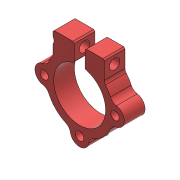
# Autodesk Inventor part: 16_022_TIBIA_PIPE_CLAMPER_R1
Saved by Autodesk Inventor 2021.2 (Build 252289000, 289)
## iProperties
Created: 2018-07-20
Part Number: 16_022_TIBIA_PIPE_CLAMPER_R1
Material: アルミニウム 6061
Document SubType Name: Modeling
Designer: student
Density: 2.7 g/cm^3
Appearance: 滑らか - 赤
Mass: 0.864961 g
Surface Area: 6.24289 cm^2
Volume: 0.320356 cm^3
Author: student
Autodesk Inventor part; units mm, degrees
ref_plane "YZ Plane" through (0, 0, 0) normal (1, 0, 0) x (0, 1, 0)
ref_plane "XZ Plane" through (0, 0, 0) normal (0, 1, 0) x (-1, 0, 0)
ref_plane "XY Plane" through (0, 0, 0) normal (0, 0, 1) x (1, 0, 0)
sketch "スケッチ1" plane through (0, 0, 0) normal (0, 1, 0) x (-1, 0, 0)
  arc A0 (-1.2381, 4.8443) -> (1.2381, 4.8443) centre (0, 0) ccw
  line L0 (1.05, 5.0865) -> (1.05, 8.0865)
  line L1 (1.3, 8.3365) -> (4.8692, 8.3365)
  line L2 (-1.05, 5.0865) -> (-1.05, 8.0865)
  line L3 (-1.3, 8.3365) -> (-4.4822, 8.3365)
  line L4 (-4.7322, 8.0865) -> (-4.7322, 4.8365)
  line L5 (0, 0) -> (0, 8.2759) construction
  arc A1 (1.05, 5.0865) -> (1.2381, 4.8443) centre (1.3, 5.0865) ccw
  arc A2 (-1.2381, 4.8443) -> (-1.05, 5.0865) centre (-1.3, 5.0865) ccw
  arc A3 (-1.7788, -7.0755) -> (1.7788, -7.0755) centre (0, -6.8) ccw
  arc A4 (-4.9679, 4.1916) -> (-5.9354, 2.6497) centre (0, 0) ccw
  arc A5 (2.6497, -5.9354) -> (5.9354, -2.6497) centre (0, 0) ccw
  line L6 (0, -6.8) -> (0, 0) construction
  arc A6 (2.6497, -5.9354) -> (1.7788, -7.0755) centre (3.2611, -7.3051) ccw
  arc A7 (-1.7788, -7.0755) -> (-2.6497, -5.9354) centre (-3.2611, -7.3051) ccw
  circle A8 centre (0, -6.8) radius 0.8
  arc A9 (5.1192, 4.3365) -> (5.3033, 3.7583) centre (6.1192, 4.3365) ccw
  arc A10 (-4.9679, 4.1916) -> (-4.7322, 4.8365) centre (-5.7322, 4.8365) ccw
  line L7 (1.05, 8.0865) -> (1.3, 8.3365)
  line L8 (-1.05, 8.0865) -> (-1.3, 8.3365)
  arc A11 (5.1192, 7.1865) -> (5.1192, 5.9865) centre (5.9192, 6.5865) ccw
  line L9 (5.1192, 8.0865) -> (5.1192, 7.1865)
  line L10 (5.1192, 5.9865) -> (5.1192, 4.3365)
  line L11 (1.05, 6.5865) -> (5.9192, 6.5865) construction
  line L12 (5.1192, 8.0865) -> (4.8692, 8.3365)
  line L13 (-4.7322, 8.0865) -> (-4.4822, 8.3365)
  arc A12 (7.0755, -1.7788) -> (7.0755, 1.7788) centre (6.8, 0) ccw
  arc A13 (6.2684, -1.7197) -> (6.2684, 1.7197) centre (0, 0) ccw construction
  arc A14 (5.9354, 2.6497) -> (5.3033, 3.7583) centre (0, 0) ccw
  circle A15 centre (6.8, 0) radius 0.8
  arc A16 (7.0755, -1.7788) -> (5.9354, -2.6497) centre (7.3051, -3.2611) ccw
  arc A17 (5.9354, 2.6497) -> (7.0755, 1.7788) centre (7.3051, 3.2611) ccw
  line L14 (6.8, 0) -> (0, 0) construction
  arc A18 (-7.0755, 1.7788) -> (-7.0755, -1.7788) centre (-6.8, 0) ccw
  circle A19 centre (-6.8, 0) radius 0.8
  arc A20 (-5.9354, -2.6497) -> (-7.0755, -1.7788) centre (-7.3051, -3.2611) ccw
  arc A21 (-7.0755, 1.7788) -> (-5.9354, 2.6497) centre (-7.3051, 3.2611) ccw
  arc A22 (-5.9354, -2.6497) -> (-2.6497, -5.9354) centre (0, 0) ccw
  arc A23 (-5.9354, 2.6497) -> (-5.9354, -2.6497) centre (0, 0) ccw construction
  point P0 (-1.05, 4.8885)
  point P1 (1.05, 4.8885)
  point P2 (1.05, 8.3365)
  point P3 (5.1192, 8.3365)
  point P4 (5.1192, 4.0055)
  point P5 (-1.05, 8.3365)
  point P6 (-4.7322, 8.3365)
  point P7 (-4.7322, 4.456)
  dimension "d0" = 5
  dimension "d1" = 2.1
  dimension "d2" = 0.25
  dimension "d8" = 6.5
  dimension "d9" = 1.8
  dimension "d11" = 1.5
  dimension "d12" = 1.6
  dimension "d13" = 1
  dimension "d14" = 4
  dimension "d15" = 3.5
  dimension "d16" = 0.25
  dimension "d17" = 0.25
  dimension "d18" = 0.25
  dimension "d19" = 0.25
  dimension "d20" = 3
  dimension "d21" = 1
  dimension "d22" = 0.8
  dimension "d23" = 0.25
  dimension "d24" = 0.25
  dimension "d25" = 0.25
  dimension "d26" = 0.25
  dimension "d27" = 1.5
  constraints: 51 point on circle, 30 end point, 24 centre point, 19 tangent, 11 point on line, 8 symmetric about line, 7 equal radius, 5 perpendicular, 4 vertical, 3 coincident, 2 horizontal, 1 collinear, 1 concentric, 1 midpoint, 5 other
  measures "d0" radius of A0
  measures "d1" distance between parallel lines of L2 L0
  measures "d2" radius of A1
  measures "d8" radius of A5
  measures "d9" radius of A3
  measures "d11" radius of A6
  measures "d12" diameter of A8
  measures "d13" radius of A9
  measures "d14" distance of point (5.119, 8.337) L10.end
  measures "d15" distance of point (-4.732, 8.337) L4.end
  measures "d16" distance of L0.end point (1.05, 8.337)
  measures "d17" distance of L1.start point (1.05, 8.337)
  measures "d18" distance of L2.end point (-1.05, 8.337)
  measures "d19" distance of L3.start point (-1.05, 8.337)
  measures "d20" distance of L0.start L0.end
  measures "d21" radius of A11
  measures "d22" distance from line of L10 L11.end
  measures "d23" distance of L9.start point (5.119, 8.337)
  measures "d24" distance of L1.end point (5.119, 8.337)
  measures "d25" distance of L4.start point (-4.732, 8.337)
  measures "d26" distance of L3.end point (-4.732, 8.337)
  measures "d27" radius of A16
extrude "押し出し1" add sketch "スケッチ1" along normal blind 4
sketch "スケッチ2" plane through (-5.1192, 0, 7.1865) normal (-1, 0, 0) x (0, 0, 1)
  circle A0 centre (-0.6, 2) radius 1
  line L0 (-0.6, 2) -> (-0.6, 4) construction
  line L1 (-2.1, 4) -> (0.9, 4) construction
  point P0 (-7.1865, 0)
  dimension "d30" = 2
  dimension "d31" = 2
  constraints: 2 end point, 1 centre point, 1 midpoint, 1 vertical
  measures "d30" distance of L0.start L0.end
  measures "d31" diameter of A0
extrude "押し出し2" cut sketch "スケッチ2" against normal blind 10
equation "\"d17\" = d16"
equation "\"d18\" = d16"
equation "\"d19\" = d18"
equation "\"d24\" = d23"
equation "\"d25\" = d23"
equation "\"d26\" = d25"
